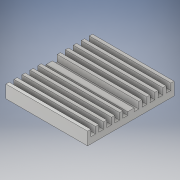
# Autodesk Inventor part: Copper Radiator
Saved by Autodesk Inventor 2019.2 (Build 232265000, 265)
## iProperties
Created: 2018-12-13
Part Number: Copper Radiator
Material: Aluminum 6061-AHC
Document SubType Name: Modeling
Designer: Petar
Density: 2.7 g/cm^3
Appearance: Aluminum - Dark
Author: Petar
Autodesk Inventor part; units mm, degrees
ref_plane "YZ Plane" through (0, 0, 0) normal (1, 0, 0) x (0, 1, 0)
ref_plane "XZ Plane" through (0, 0, 0) normal (0, 1, 0) x (-1, 0, 0)
ref_plane "XY Plane" through (0, 0, 0) normal (0, 0, 1) x (1, 0, 0)
sketch "Sketch1" plane through (0, 0, 0) normal (0, 1, 0) x (-1, 0, 0)
  line L0 (12.75, 13.5) -> (-12.75, 13.5)
  line L1 (-12.75, 13.5) -> (-12.75, -13.5)
  line L2 (-12.75, -13.5) -> (12.75, -13.5)
  line L3 (12.75, -13.5) -> (12.75, 13.5)
  line L4 (0, 13.5) -> (0, -13.5) construction
  line L5 (12.75, 0) -> (-12.75, 0) construction
  point P0 (0, 0)
  point P1 (0, 0)
  dimension "d0" = 25.5
  dimension "d1" = 27
  constraints: 12 end point, 5 midpoint, 2 parallel, 1 coincident, 1 horizontal, 1 perpendicular
  measures "d0" distance of L2.end L1.end
  measures "d1" distance of L1.end L0.end
extrude "Extrusion1" add sketch "Sketch1" along normal blind 4
sketch "Sketch2" plane through (-12.75, 0, -13.5) normal (-1, 0, 0) x (0, 0, 1)
  line L0 (0, 0) -> (27, 0) projected
  line L1 (0, 0) -> (0, 4) projected
  line L2 (27, 4) -> (0, 4) projected
  line L3 (1, 4) -> (2.5, 4)
  line L4 (2.5, 4) -> (2.5, 2)
  line L5 (2.5, 2) -> (1, 2)
  line L6 (1, 2) -> (1, 4)
  line L7 (13.5, 0) -> (13.5, 4) construction
  line L8 (3.5, 4) -> (5, 4)
  line L9 (5, 4) -> (5, 2)
  line L10 (5, 2) -> (3.5, 2)
  line L11 (3.5, 2) -> (3.5, 4)
  line L12 (6, 4) -> (7.5, 4)
  line L13 (7.5, 4) -> (7.5, 2)
  line L14 (7.5, 2) -> (6, 2)
  line L15 (6, 2) -> (6, 4)
  line L16 (8.5, 4) -> (10, 4)
  line L17 (10, 4) -> (10, 2)
  line L18 (10, 2) -> (8.5, 2)
  line L19 (8.5, 2) -> (8.5, 4)
  line L20 (26, 4) -> (24.5, 4)
  line L21 (24.5, 4) -> (24.5, 2)
  line L22 (24.5, 2) -> (26, 2)
  line L23 (26, 2) -> (26, 4)
  line L24 (23.5, 4) -> (22, 4)
  line L25 (22, 4) -> (22, 2)
  line L26 (22, 2) -> (23.5, 2)
  line L27 (23.5, 2) -> (23.5, 4)
  line L28 (21, 4) -> (19.5, 4)
  line L29 (19.5, 4) -> (19.5, 2)
  line L30 (19.5, 2) -> (21, 2)
  line L31 (21, 2) -> (21, 4)
  line L32 (18.5, 4) -> (17, 4)
  line L33 (17, 4) -> (17, 2)
  line L34 (17, 2) -> (18.5, 2)
  line L35 (18.5, 2) -> (18.5, 4)
  line L36 (0, 4) -> (27, 4) projected
  line L37 (11, 4) -> (12.5, 4)
  line L38 (12.5, 3) -> (12.5, 2)
  line L39 (12.5, 2) -> (11, 2)
  line L40 (11, 2) -> (11, 4)
  line L41 (16, 4) -> (14.5, 4)
  line L42 (14.5, 3) -> (14.5, 2)
  line L43 (14.5, 2) -> (16, 2)
  line L44 (16, 2) -> (16, 4)
  line L45 (12.5, 3) -> (13.5, 3)
  line L46 (13.5, 3) -> (14.5, 3)
  line L47 (12.5, 4) -> (14.5, 4)
  dimension "d5" = 1
  dimension "d6" = 1.5
  dimension "d7" = 1.5
  dimension "d8" = 1
  dimension "d9" = 1.5
  dimension "d10" = 1
  dimension "d12" = 2
  dimension "d13" = 1.5
  dimension "d14" = 1
  dimension "d17" = 1.5
  dimension "d18" = 1
  constraints: 88 end point, 20 symmetric about line, 10 parallel, 7 horizontal, 7 point on line, 5 perpendicular, 3 collinear, 1 midpoint
  measures "d5" distance between parallel lines of L1 L6
  measures "d6" distance of L9.end L10.end
  measures "d7" distance of L13.end L14.end
  measures "d8" distance between parallel lines of L4 L11
  measures "d9" distance of L4.end L5.end
  measures "d10" distance between parallel lines of L9 L15
  measures "d12" distance between parallel lines of L0 L5
  measures "d13" distance of L17.end L18.end
  measures "d14" distance between parallel lines of L19 L13
  measures "d17" distance of L38.end L39.end
  measures "d18" distance between parallel lines of L40 L17
extrude "Extrusion3" cut sketch "Sketch2" against normal through all
body "Solid1"
